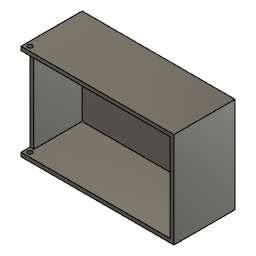
UselessBoxBottom v3 (Autodesk Fusion 360 design; units mm, degrees)
Autodesk Fusion 360 part; units mm, degrees
note: some values were not read from the file. Set by a fixed rule: which sketch regions a step uses.
sketch "Sketch1" plane through (0, 0, 0) normal (0, 0, 1) x (1, 0, 0)
  line L0 (0, 0) -> (203.2, 0)
  line L1 (203.2, 0) -> (203.2, 127)
  line L2 (203.2, 127) -> (0, 127)
  line L3 (0, 127) -> (0, 0)
  dimension "d1" = 203.2
  dimension "d2" = 127
  constraint horizontal L0
  constraint vertical L1
  constraint horizontal L2
  constraint vertical L3
  constraint coincident L0.start L3.end
  measures "d1" distance of L0.start L0.end
  measures "d2" distance of L0.start L2.end
extrude "Extrude1" add sketch "Sketch1" along normal blind 5
sketch "Sketch2" plane through (0, 0, 5) normal (0, 0, 1) x (1, 0, 0)
  line L0 (0, 127) -> (0, 0)
  line L1 (0, 0) -> (203.2, 0)
  line L2 (203.2, 0) -> (203.2, 127)
  line L3 (203.2, 127) -> (0, 127)
  line L4 (0, 127) -> (5, 127)
  line L5 (0, 122) -> (0, 127)
  line L6 (203.2, 0) -> (198.2, 0)
  line L7 (203.2, 5) -> (203.2, 0)
  line L8 (5, 122) -> (198.2, 122)
  line L9 (198.2, 122) -> (198.2, 5)
  line L10 (198.2, 5) -> (5, 5)
  line L11 (5, 5) -> (5, 122)
  constraint horizontal L4
  constraint vertical L5
  constraint coincident L0.start L3.end
  constraint horizontal L6
  constraint vertical L7
  constraint coincident L1.end L2.start
  constraint horizontal L8
  constraint vertical L9
  constraint horizontal L10
  constraint vertical L11
extrude "Extrude2" add sketch "Sketch2" along normal blind 76.2
sketch "Sketch3" plane through (0, 0, 81.2) normal (0, 0, 1) x (1, 0, 0)
  line L0 (198.2, 5) -> (5, 5)
  line L1 (5, 5) -> (5, 122)
  line L2 (5, 122) -> (198.2, 122)
  line L3 (198.2, 122) -> (198.2, 5)
  line L4 (203.2, 127) -> (0, 127)
  line L5 (0, 127) -> (0, 0)
  line L6 (0, 0) -> (203.2, 0)
  line L7 (203.2, 0) -> (203.2, 127)
  line L8 (5, 122) -> (0, 122)
  line L9 (0, 122) -> (0, 5)
  line L10 (0, 5) -> (5, 5)
  line L11 (5, 5) -> (5, 122)
  constraint horizontal L8
  constraint vertical L9
  constraint horizontal L10
  constraint vertical L11
  constraint coincident L5 L9.end
  constraint coincident L1.end L2.start
extrude "Extrude3" cut sketch "Sketch3" against normal blind 10 contours L1 L5 L8 L9 L10 L11
sketch "Sketch4" plane through (0, 0, 0) normal (0, -1, 0) x (1, 0, 0)
  line L0 (0, 0) -> (203.2, 0)
  line L1 (203.2, 0) -> (203.2, 81.2)
  line L2 (203.2, 81.2) -> (0, 81.2)
  line L3 (0, 81.2) -> (0, 0)
  line L4 (0, 81.2) -> (6, 81.2)
  line L5 (6, 81.2) -> (6, 75.2)
  line L6 (6, 75.2) -> (0, 75.2)
  line L7 (0, 75.2) -> (0, 81.2)
  circle A0 centre (6, 75.2) radius 3
  line L8 (203.2, 0) -> (183.2, 0)
  line L9 (183.2, 0) -> (183.2, 20)
  line L10 (183.2, 20) -> (203.2, 20)
  line L11 (203.2, 20) -> (203.2, 0)
  circle A1 centre (183.2, 20) radius 5
  line L12 (183.2, 20) -> (158.2, 20)
  line L13 (158.2, 20) -> (158.2, 0)
  line L14 (158.2, 0) -> (183.2, 0)
  line L15 (183.2, 0) -> (183.2, 20)
  circle A2 centre (158.2, 20) radius 10
  dimension "d13" = 6
  dimension "d14" = 6
  dimension "d15" = 6
  dimension "d16" = 20
  dimension "d17" = 20
  dimension "d18" = 10
  dimension "d19" = 25
  dimension "d20" = 20
  constraint horizontal L4
  constraint vertical L5
  constraint horizontal L6
  constraint vertical L7
  constraint coincident L2.end L3.start
  constraint coincident L5.end L6.start
  constraint horizontal L8
  constraint vertical L9
  constraint horizontal L10
  constraint vertical L11
  constraint coincident L0.end L1.start
  constraint coincident L9.end L10.start
  constraint horizontal L12
  constraint vertical L13
  constraint horizontal L14
  constraint vertical L15
  constraint coincident L12.end L13.start
  measures "d13" distance of L2.end L4.end
  measures "d14" distance of L2.end L6.end
  measures "d15" diameter of A0
  measures "d16" distance of L0.end L8.end
  measures "d17" distance of L0.end L10.end
  measures "d18" diameter of A1
  measures "d19" distance of L9.end L12.end
  measures "d20" diameter of A2
extrude "Extrude4" cut sketch "Sketch4" against normal blind 5 contours L12 L13 A2 | L12 L13 A2 | L5 L6 A0 | L5 L6 A0 | L9 A1 L12 L15 | L9 L10 A1 L15 | L10 A1 L12
extrude "Extrude5" cut 1 faces at (3.3333, 44, 71.2) along direction (0, 0, -1) blind 2
sketch "Sketch5" plane through (0, 127, 0) normal (0, 1, 0) x (-1, 0, 0)
  line L0 (-203.2, 0) -> (0, 0)
  line L1 (0, 0) -> (0, 81.2)
  line L2 (0, 81.2) -> (-203.2, 81.2)
  line L3 (-203.2, 81.2) -> (-203.2, 0)
  line L4 (0, 81.2) -> (-6, 81.2)
  line L5 (-6, 81.2) -> (-6, 75.2)
  line L6 (-6, 75.2) -> (0, 75.2)
  line L7 (0, 75.2) -> (0, 81.2)
  circle A0 centre (-6, 75.2) radius 3
  dimension "d25" = 6
  dimension "d26" = 6
  dimension "d27" = 6
  constraint horizontal L4
  constraint vertical L5
  constraint horizontal L6
  constraint vertical L7
  constraint coincident L1.end L2.start
  constraint coincident L5.end L6.start
  measures "d25" distance of L1.end L4.end
  measures "d26" distance of L1.end L6.end
  measures "d27" diameter of A0
extrude "Extrude6" cut sketch "Sketch5" against normal blind 5 contours L5 L6 A0 | L5 L6 A0
sketch "Sketch6" plane through (0, 0, 5) normal (0, 0, 1) x (1, 0, 0)
  line L0 (198.2, 5) -> (198.2, 122)
  line L1 (198.2, 122) -> (5, 122)
  line L2 (5, 122) -> (5, 5)
  line L3 (5, 5) -> (198.2, 5)
  line L4 (60, 93.0795) -> (150.2102, 93.0795) construction
  line L5 (150.2102, 93.0795) -> (150.2102, 120) construction
  line L6 (150.2102, 120) -> (60, 120) construction
  line L7 (60, 120) -> (60, 93.0795) construction
  dimension "d30" = 5
  text T0 "Sam Rutschilling 2022" font "Arial" height 5 align left top in box 90.2102 x 26.9205 at (60, 93.0795) x (1, 0) y (0, 1) spacing 1
extrude "Extrude7" add sketch "Sketch6" along normal blind 1 text T0
